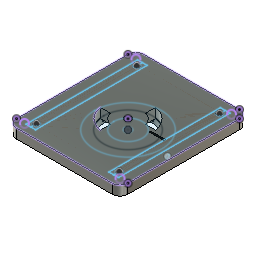
rotary base 1 v7 (Autodesk Fusion 360 design; units mm, degrees)
Autodesk Fusion 360 part; units mm, degrees
note: some values were not read from the file. Chosen so that the rebuilt part matches the saved one: which face or edge a step refers to. Set by a fixed rule: which sketch regions a step uses.
sketch "mouting rings" plane through (0, 0, 84.5) normal (0, 0, 1) x (-1, 0, 0)
  circle A0 centre (0, 0) radius 19.05
  circle A1 centre (0, 0) radius 30
  circle A2 centre (0, 0) radius 18
  circle A3 centre (0, 0) radius 30.5
  circle A4 centre (0, 0) radius 42
  circle A5 centre (0, 0) radius 4.25
  dimension "d1" = 61
  dimension "d16" = 8.5
  constraint coincident A0.centre A1.centre
  measures "d1" diameter of A3
  measures "d16" diameter of A5
extrude "Extrude1" add sketch "mouting rings" against normal blind 8 contours A2 | A4 | A5 makes body 1 at (-4.9925, -1.2634, 84.5) makes body 2 at (-37.8967, 3.6019, 84.5)
ref_plane "WorkPlane1" through (49.5, 0, 69.7065) normal (1, 0, 0) x (0, -1, 0)
sketch "mounting point holes" plane through (49.5, 0, 0) normal (1, 0, 0) x (0, 1, 0)
  circle A0 centre (0, 80.5) radius 2.2
  dimension "d5" = 4.4
  measures "d5" diameter of A0
extrude "Extrude2" cut sketch "mounting point holes" against normal blind 49 bodies 1 2
pattern_circular "C-Pattern1" count 4 over 360 about axis through (0, 0, 84.5) along (0, 0, -1) of "Extrude2"
sketch "base" plane through (0, 0, 84.5) normal (0, 0, 1) x (-1, 0, 0)
  circle A0 centre (0, 0) radius 4.25
  line L0 (-5, -24.5) -> (-5, -17.2916)
  line L1 (-5, -24.5) -> (-5, -29.8339)
  line L2 (24.5, 5) -> (17.2916, 5)
  line L3 (24.8332, 5) -> (29.8339, 5)
  line L4 (5, 24.5) -> (5, 29.8339)
  line L5 (5, 24.5) -> (5, 17.2916)
  line L6 (-24.5, -5) -> (-17.2916, -5)
  line L7 (-24.8332, -5) -> (-29.8339, -5)
  arc A1 (17.2916, 5) -> (5, 17.2916) centre (0, 0) ccw
  arc A2 (29.8339, 5) -> (5, 29.8339) centre (0, 0) ccw
  arc A3 (-17.2916, -5) -> (-5, -17.2916) centre (0, 0) ccw
  arc A4 (-29.8339, -5) -> (-5, -29.8339) centre (0, 0) ccw
  line L8 (24.8332, 5) -> (24.5, 5)
  line L9 (-24.5, -5) -> (-24.8332, -5)
  line L10 (70, 0) -> (70, -70)
  line L11 (70, 0) -> (70, 70)
  line L12 (-5, 80) -> (60, 80)
  line L13 (-5, 80) -> (-60, 80)
  line L14 (-70, 0) -> (-70, 70)
  line L15 (0, -80) -> (60, -80)
  line L16 (0, -80) -> (-60, -80)
  line L17 (-70, -70) -> (-70, 0)
  arc A5 (60, -80) -> (70, -70) centre (60, -70) ccw
  arc A6 (-70, -70) -> (-60, -80) centre (-60, -70) ccw
  arc A7 (70, 70) -> (60, 80) centre (60, 70) ccw
  arc A8 (-60, 80) -> (-70, 70) centre (-60, 70) ccw
  point P0 (95, -95)
  point P1 (-95, -95)
  point P2 (95, 95)
  dimension "d12" = 190
  dimension "d13" = 190
  dimension "d15" = 8.5
  dimension "d55" = 10
  dimension "d56" = 10
  dimension "d57" = 10
  dimension "d58" = 10
  constraint coincident A0.centre A1.centre
  constraint parallel L2 L8
  constraint perpendicular L11 L12
  constraint perpendicular L13 L14
  constraint perpendicular L10 L15
  constraint tangent L15 A5
  constraint tangent L10 A5
  constraint tangent L16 A6
  constraint tangent L17 A6
  constraint tangent L11 A7
  constraint tangent L12 A7
  constraint tangent L13 A8
  constraint tangent L14 A8
  measures "d12" distance of P0 P1
  measures "d13" distance of P0 P2
  measures "d15" diameter of A0
  measures "d55" radius of A5
  measures "d56" radius of A6
  measures "d57" radius of A7
  measures "d58" radius of A8
extrude "Extrude3" cut sketch "base" against normal blind 8 contours A0 bodies 1
extrude "Extrude4" add sketch "base" along normal blind 12 contours L0 L1 L6 L7 A3 A4 L9 | L2 L3 L4 L5 A1 A2 L8 | L10 L11 L12 L13 L14 L15 L16 L17 A5 A6 A7 A8 bodies 1 2
split "Split1" by plane through (0, 0, 84.5) normal (0, 0, -1) bodies 1 makes body 3 at (-13.3338, 1.1054, 76.5) makes body 4 at (-37.8967, 3.6019, 76.5)
delete_body "RemoveBody1" bodies 1
extrude "Extrude5" add sketch "base" along normal blind 12 bodies 3 4
sketch "superstructure mouting holes" plane through (0, 0, 96.5) normal (0, 0, 1) x (-1, 0, 0)
  line L0 (-29.8339, -5) -> (-17.2916, -5)
  arc A0 (-17.2916, -5) -> (-5, -17.2916) centre (0, 0) ccw
  line L1 (-5, -17.2916) -> (-5, -29.8339)
  arc A1 (-29.8339, -5) -> (-5, -29.8339) centre (0, 0) ccw
  line L2 (29.8339, 5) -> (17.2916, 5)
  arc A2 (17.2916, 5) -> (5, 17.2916) centre (0, 0) ccw
  line L3 (5, 17.2916) -> (5, 29.8339)
  circle A3 centre (0, 0) radius 4.25
  line L4 (-46, 0) -> (-46, 70)
  line L5 (-46, 0) -> (-46, -70)
  line L6 (46, 0) -> (46, -70)
  line L7 (46, 0) -> (46, 70)
  line L8 (-46, 70) -> (-58, 70)
  line L9 (46, 70) -> (58, 70)
  line L10 (58, 70) -> (58, -70)
  line L11 (58, -70) -> (46, -70)
  line L12 (-46, -70) -> (-58, -70)
  line L13 (-58, -70) -> (-58, 70)
  line L14 (52, -70) -> (52, -63)
  line L15 (-52, -70) -> (-52, -63)
  line L16 (-52, 70) -> (-52, 63)
  line L17 (52, 70) -> (52, 63)
  arc A4 (29.8339, 5) -> (5, 29.8339) centre (0, 0) ccw
  circle A5 centre (52, 63) radius 3.25
  circle A6 centre (-52, 63) radius 3.25
  circle A7 centre (52, -63) radius 3.25
  circle A8 centre (-52, -63) radius 3.25
  line L18 (70, -70) -> (70, 70)
  line L19 (60, 80) -> (-60, 80)
  line L20 (-60, -80) -> (60, -80)
  line L21 (-70, 70) -> (-70, -70)
  arc A9 (-60, 80) -> (-70, 70) centre (-60, 70) ccw
  arc A10 (-70, -70) -> (-60, -80) centre (-60, -70) ccw
  arc A11 (60, -80) -> (70, -70) centre (60, -70) ccw
  arc A12 (70, 70) -> (60, 80) centre (60, 70) ccw
  dimension "d28" = 46
  dimension "d29" = 46
  dimension "d30" = 70
  dimension "d31" = 70
  dimension "d32" = 70
  dimension "d33" = 70
  dimension "d34" = 12
  dimension "d35" = 12
  dimension "d36" = 12
  dimension "d46" = 6.5
  dimension "d47" = 6.5
  dimension "d48" = 6.5
  dimension "d49" = 6.5
  constraint vertical L5
  constraint perpendicular L4 L8
  constraint perpendicular L7 L9
  constraint perpendicular L9 L10
  constraint perpendicular L6 L11
  constraint perpendicular L5 L12
  constraint perpendicular L8 L13
  constraint midpoint L11 L14.start
  constraint perpendicular L11 L14
  constraint midpoint L12 L15.start
  constraint perpendicular L12 L15
  constraint midpoint L8 L16.start
  constraint perpendicular L8 L16
  constraint midpoint L9 L17.start
  constraint perpendicular L9 L17
  constraint coincident L17.end A5.centre
  constraint coincident L16.end A6.centre
  constraint coincident L14.end A7.centre
  constraint coincident L15.end A8.centre
  measures "d28" distance of A0.centre L4.start
  measures "d29" distance of A0.centre L6.start
  measures "d30" distance of L4.start L4.end
  measures "d31" distance of L4.start L5.end
  measures "d32" distance of L6.start L6.end
  measures "d33" distance of L6.start L7.end
  measures "d34" distance of L4.end L8.end
  measures "d35" distance of L7.end L9.end
  measures "d36" distance of L5.end L12.end
  measures "d46" diameter of A5
  measures "d47" diameter of A6
  measures "d48" diameter of A7
  measures "d49" diameter of A8
sketch "Sketch6" plane through (0, 0, 96.5) normal (0, 0, 1) x (-1, 0, 0)
  line L0 (-46, 1) -> (-28, 1)
  line L1 (-28, 1) -> (-27.5, 1)
  line L2 (-27.5, 1) -> (-27.5, -1)
  line L3 (-27.5, -1) -> (-46, -1)
  line L4 (-46, 1) -> (-46, -1)
  constraint perpendicular L2 L3
  constraint perpendicular L0 L4
extrude "Extrude6" cut sketch "Sketch6" against normal blind 1 bodies 3
extrude "Extrude7" cut sketch "superstructure mouting holes" against normal blind 12 contours A5 | A6 | A7 | A8 bodies 3
sketch "Sketch7" plane through (0, 0, 84.5) normal (0, 0, -1) x (1, 0, 0)
  circle A0 centre (52, -63) radius 3.25
  circle A1 centre (52, 63) radius 3.25
  circle A2 centre (-52, -63) radius 3.25
  circle A3 centre (-52, 63) radius 3.25
  line L0 (60, 80) -> (-60, 80)
  arc A4 (-60, 80) -> (-70, 70) centre (-60, 70) ccw
  line L1 (-70, 70) -> (-70, -70)
  arc A5 (-70, -70) -> (-60, -80) centre (-60, -70) ccw
  line L2 (-60, -80) -> (60, -80)
  arc A6 (60, -80) -> (70, -70) centre (60, -70) ccw
  line L3 (70, -70) -> (70, 70)
  arc A7 (70, 70) -> (60, 80) centre (60, 70) ccw
  circle A8 centre (0, 0) radius 42
  line L4 (-46.9, 65.9445) -> (-52, 68.889)
  line L5 (-52, 68.889) -> (-57.1, 65.9445)
  line L6 (-57.1, 65.9445) -> (-57.1, 60.0555)
  line L7 (-57.1, 60.0555) -> (-52, 57.111)
  line L8 (-52, 57.111) -> (-46.9, 60.0555)
  line L9 (-46.9, 60.0555) -> (-46.9, 65.9445)
  line L10 (-46.9, -60.0555) -> (-52, -57.111)
  line L11 (-52, -57.111) -> (-57.1, -60.0555)
  line L12 (-57.1, -60.0555) -> (-57.1, -65.9445)
  line L13 (-57.1, -65.9445) -> (-52, -68.889)
  line L14 (-52, -68.889) -> (-46.9, -65.9445)
  line L15 (-46.9, -65.9445) -> (-46.9, -60.0555)
  line L16 (57.1, 65.9445) -> (52, 68.889)
  line L17 (52, 68.889) -> (46.9, 65.9445)
  line L18 (46.9, 65.9445) -> (46.9, 60.0555)
  line L19 (46.9, 60.0555) -> (52, 57.111)
  line L20 (52, 57.111) -> (57.1, 60.0555)
  line L21 (57.1, 60.0555) -> (57.1, 65.9445)
  line L22 (57.1, -60.0555) -> (52, -57.111)
  line L23 (52, -57.111) -> (46.9, -60.0555)
  line L24 (46.9, -60.0555) -> (46.9, -65.9445)
  line L25 (46.9, -65.9445) -> (52, -68.889)
  line L26 (52, -68.889) -> (57.1, -65.9445)
  line L27 (57.1, -65.9445) -> (57.1, -60.0555)
  point P0 (-52, 63)
  point P1 (-52, -63)
  point P2 (52, 63)
  point P3 (52, -63)
  dimension "d59" = 5.1
  dimension "d60" = 5.1
  dimension "d61" = 5.1
  dimension "d62" = 5.1
  constraint coincident P0 A3.centre
  constraint coincident P1 A2.centre
  constraint coincident A1.centre P2
  constraint coincident P3 A0.centre
  measures "d59" distance of P0 L9
  measures "d60" distance of P1 L15
  measures "d61" distance of P2 L21
  measures "d62" distance of P3 L27
extrude "Extrude8" cut sketch "Sketch7" against normal blind 4 contours L4 L5 L6 L7 L8 L9 | L10 L11 L12 L13 L14 L15 | L16 L17 L18 L19 L20 L21 | L22 L23 L24 L25 L26 L27 bodies 3
equation "heatset_5m_width_top = 6.8 mm"
equation "heatset_5m_width_BOT = 6.15 mm"
